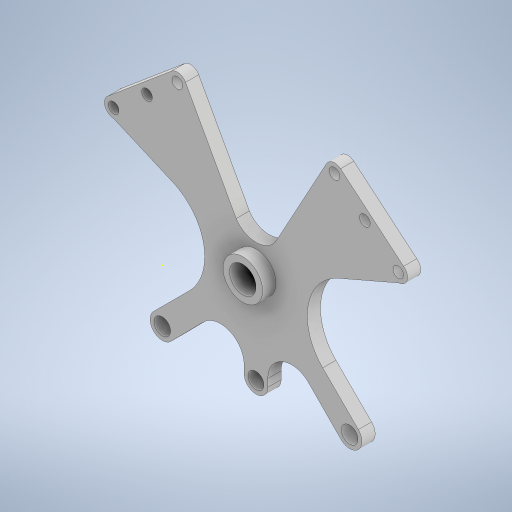
# Autodesk Inventor part: batteryclip2
Saved by Autodesk Inventor 2023 (Build 270158000, 158)
## iProperties
Created: 2023-02-09
Part Number: batteryclip2
Material: Generic
Document SubType Name: Modeling
Designer: zayda
Density: 1 g/cm^3
Appearance: Default
Author: zayda
Autodesk Inventor part; units mm, degrees
ref_plane "YZ Plane" through (0, 0, 0) normal (1, 0, 0) x (0, 1, 0)
ref_plane "XZ Plane" through (0, 0, 0) normal (0, 1, 0) x (-1, 0, 0)
ref_plane "XY Plane" through (0, 0, 0) normal (0, 0, 1) x (1, 0, 0)
sketch "Sketch2" plane through (0, 0, 0) normal (0, 0, 1) x (1, 0, 0)
  circle A0 centre (-18.4063, 42.5332) radius 2
  circle A1 centre (-5.7666, 53.1392) radius 2
  circle A2 centre (5.7241, 62.781) radius 2
  circle A3 centre (0, -20) radius 3.1284
  arc A4 (35.5, -17) -> (35.5, -23) centre (35.5, -20) ccw
  circle A5 centre (-18.4063, 42.5332) radius 3.5
  circle A6 centre (5.7241, 62.781) radius 3.5
  line L0 (-18.4063, 42.5332) -> (-5.7666, 53.1392)
  line L1 (-5.7666, 53.1392) -> (5.7241, 62.781)
  line L2 (-20.4063, 45.4055) -> (3.4731, 65.4612)
  line L3 (-15.925, 40.0648) -> (7.9726, 60.0989)
  line L4 (-5.7666, 53.1392) -> (35.5, 15.6275)
  line L5 (-18.5849, 39.0378) -> (4.0074, 29.2589)
  circle A7 centre (0, -20) radius 4.6284
  arc A8 (35.5, -15.5) -> (35.5, -24.5) centre (35.5, -20) ccw
  line L6 (35.5, 15.6275) -> (0, -20)
  line L7 (-3.2742, -16.7286) -> (10.2111, -3.2315)
  line L8 (31, -17.1135) -> (31, -20)
  line L9 (3.2938, -23.2516) -> (15.5951, -10.7907)
  arc A9 (10.2111, -3.2315) -> (4.0074, 29.2589) centre (-3.9371, 10.9045) ccw
  arc A10 (31, -17.1135) -> (15.5951, -10.7907) centre (22, -17.1135) ccw
  line L10 (27.9905, 29.3594) -> (8.7949, 64.4604)
  circle A11 centre (89.4063, 42.5332) radius 2
  circle A12 centre (76.7666, 53.1392) radius 2
  circle A13 centre (65.2759, 62.781) radius 2
  circle A14 centre (71, -20) radius 3.1284
  arc A15 (35.5, -23) -> (35.5, -17) centre (35.5, -20) ccw
  circle A16 centre (89.4063, 42.5332) radius 3.5
  circle A17 centre (65.2759, 62.781) radius 3.5
  line L11 (89.4063, 42.5332) -> (76.7666, 53.1392)
  line L12 (76.7666, 53.1392) -> (65.2759, 62.781)
  line L13 (91.4063, 45.4055) -> (67.5269, 65.4612)
  line L14 (86.925, 40.0648) -> (63.0274, 60.0989)
  line L15 (76.7666, 53.1392) -> (35.5, 15.6275)
  line L16 (89.5849, 39.0378) -> (66.9926, 29.2589)
  circle A18 centre (71, -20) radius 4.6284
  arc A19 (35.5, -24.5) -> (35.5, -15.5) centre (35.5, -20) ccw
  line L17 (35.5, 15.6275) -> (71, -20)
  line L18 (74.2742, -16.7286) -> (60.7889, -3.2315)
  line L19 (40, -17.1135) -> (40, -20)
  line L20 (67.7062, -23.2516) -> (55.4049, -10.7907)
  arc A20 (66.9926, 29.2589) -> (60.7889, -3.2315) centre (74.9371, 10.9045) ccw
  arc A21 (55.4049, -10.7907) -> (40, -17.1135) centre (49, -17.1135) ccw
  line L21 (43.0095, 29.3594) -> (62.2051, 64.4604)
  arc A22 (27.9905, 29.3594) -> (43.0095, 29.3594) centre (35.5, 34.3477) ccw
  line L22 (0, -20) -> (6.5038, -20)
  line L23 (31, -20) -> (35.5, -20)
  line L24 (71, -20) -> (64.4962, -20)
  line L25 (40, -20) -> (35.5, -20)
  circle A23 centre (35.5, 15.6275) radius 5
  point P0 (86, -15)
  point P1 (105.5095, 35.5477)
  point P2 (56.8662, 76.3642)
  point P3 (31, 11.1114)
  point P4 (40, 11.1114)
  dimension "d40" = 7
  dimension "d41" = 7
  dimension "d42" = 11.4907
  dimension "d43" = 16.5
  dimension "d44" = 4
  dimension "d45" = 1.5
  dimension "d46" = 24.1304
  dimension "d47" = 1.5
  dimension "d48" = 1.5
  dimension "d49" = 1.5
  dimension "d51" = 20
  dimension "d52" = 9
  dimension "d54" = 9.2569
  dimension "d55" = 9.0153
  dimension "d56" = 4.5
  dimension "d57" = 0.026
  dimension "d58" = 0.026
  dimension "d59" = 63.405
  dimension "d60" = 5.025
  dimension "d61" = 97.729
  dimension "d62" = 5.369
  dimension "d63" = 5.103
  dimension "d65" = 78.673
  dimension "d66" = 21.327
  dimension "d67" = 94.897
  dimension "d68" = 94.631
  dimension "d69" = 2.271
  dimension "d70" = 94.975
  dimension "d71" = 16.595
  dimension "d72" = 100.026
  dimension "d73" = 0.026
  dimension "d74" = 4.9997
  dimension "d75" = 1.5216
  dimension "d76" = 9.5286
  dimension "d77" = 59.0451
  dimension "d78" = 32.3508
  dimension "d79" = 65.5095
  dimension "d80" = 81.4761
  dimension "d81" = 3.4859
  dimension "d82" = 3.4859
  dimension "d83" = 46.2625
  dimension "d84" = 49.7327
  dimension "d85" = 3.5
  dimension "d86" = 4.9997
  dimension "d87" = 8.5066
  dimension "d88" = 39.9151
  dimension "d89" = 40.9208
  dimension "d90" = 79.1063
  dimension "d91" = 80.2554
  dimension "d92" = 84.8517
  dimension "d93" = 86.0007
  dimension "d94" = 10
  constraints: 52 end point, 32 point on circle, 24 centre point, 19 tangent, 12 point on line, 9 equal radius, 5 coincident, 2 horizontal, 2 symmetric about line, 1 collinear, 1 parallel
  measures "d40" diameter of A5
  measures "d41" diameter of A6
  measures "d42" horizontal distance of L0.end L1.end
  measures "d43" distance of L0.start L0.end
  measures "d44" diameter of A1
  measures "d45" radial gap between concentric circles of A6 A2
  measures "d46" horizontal distance of L0.start L1.end
  measures "d47" radial gap between concentric circles of A5 A0
  measures "d48" radial gap between concentric circles of A3 A7
  measures "d49" radial gap between concentric circles of A4 A8
  measures "d51" radius of A9
  measures "d52" radius of A10
  measures "d54" diameter of A18
  measures "d55" radius of A22
  measures "d56" radius of A19
  measures "d57" angle of L11 L13
  measures "d58" angle of L14 L11
  measures "d59" angle of L11 L16
  measures "d60" angle of L11 L18
  measures "d61" angle of L11 L15
  measures "d62" angle of L11 L20
  measures "d63" angle of L11 L17
  measures "d65" angle of L11 L21
  measures "d66" angle of L11 L10
  measures "d67" angle of L11 L6
  measures "d68" angle of L11 L9
  measures "d69" angle of L11 L4
  measures "d70" angle of L11 L7
  measures "d71" angle of L11 L5
  measures "d72" angle of L3 L11
  measures "d73" angle of L12 L13
  measures "d74" distance from line of point (105.509, 35.548) L11
  measures "d75" distance from line of point (105.509, 35.548) L13
  measures "d76" distance from line of point (105.509, 35.548) L16
  measures "d77" distance from line of point (105.509, 35.548) L18
  measures "d78" distance from line of point (105.509, 35.548) L15
  measures "d79" distance from line of point (105.509, 35.548) L19
  measures "d80" distance from line of point (105.509, 35.548) L3
  measures "d81" distance from line of L13.start L11
  measures "d82" distance from line of L14.start L11
  measures "d83" distance from line of point (86, -15) L11
  measures "d84" distance from line of point (86, -15) L13
  measures "d85" distance from line of L14.end L11
  measures "d86" distance from line of point (56.866, 76.364) L11
  measures "d87" distance from line of point (56.866, 76.364) L14
  measures "d88" distance from line of L21.start L11
  measures "d89" distance from line of A22.centre L11
  measures "d90" distance from line of A8.start L11
  measures "d91" distance from line of A4.start L11
  measures "d92" distance from line of A4.end L11
  measures "d93" distance from line of A8.end L11
  measures "d94" diameter of A23
extrude "Extrusion1" add sketch "Sketch2" along normal blind 5 contours A5 | A5 L2 A6 L1 A1 L0 | L0 A1 L4 L3 A5 | L3 L4 A23 L6 A7 L7 A9 L5 A5 | A6 | L1 A6 L3 L4 A1 | L3 A6 L10 A22 L21 A17 L14 L15 A23 L4 | L15 L14 A16 L16 A20 L18 A18 L17 A23 | A23 L17 A18 L24 L20 A21 L19 A19 A8 L8 A10 L9 L22 A7 L6 | A7 L6 A3 L22 | L15 A12 L11 A16 L14 | L14 A17 L12 A12 L15 | A7 L22 A3 L6 | A7 L22 L9 | A17 | L17 A14 L24 A18 | A18 L24 A14 L17 | A16 | L13 A16 L11 A12 L12 A17 | A18 L20 L24 | L23 A4 A15 L25 A19 A8 | A8 A19 L25 A15 A4 L23
sketch "Sketch3" plane through (0, 0, 5) normal (0, 0, 1) x (1, 0, 0)
  point P0 (0, 0)
sketch "Sketch4" plane through (0, 0, 5) normal (0, 0, 1) x (1, 0, 0)
  circle A0 centre (35.5, 15.6275) radius 5 projected
  circle A1 centre (35.5, 15.6275) radius 7.5
  point P0 (0, 0)
  dimension "d97" = 15
  constraints: 1 centre point, 1 coincident
  measures "d97" diameter of A1
extrude "Extrusion2" add sketch "Sketch4" along normal blind 5
body "Solid1"
